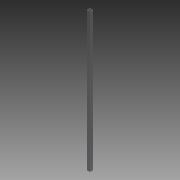
# Autodesk Inventor part: Square
Saved by Autodesk Inventor 2015 SP1 (Build 190203100, 203)
## iProperties
Created: 2015-02-01
Part Number: Square
Material: Aluminum
Document SubType Name: Modeling
Designer: Brian
Density: 2.7 g/cm^3
Appearance: Semi-Polished
Author: Brian
Autodesk Inventor part; units mm, degrees
ref_plane "YZ Plane" through (0, 0, 0) normal (1, 0, 0) x (0, 1, 0)
ref_plane "XZ Plane" through (0, 0, 0) normal (0, 1, 0) x (-1, 0, 0)
ref_plane "XY Plane" through (0, 0, 0) normal (0, 0, 1) x (1, 0, 0)
sketch "Sketch1" plane through (0, 0, 0) normal (0, 1, 0) x (-1, 0, 0)
  line L0 (12.7, -12.7) -> (-12.7, -12.7)
  line L1 (-12.7, -12.7) -> (-12.7, 12.7)
  line L2 (-12.7, 12.7) -> (12.7, 12.7)
  line L3 (12.7, 12.7) -> (12.7, -12.7)
  line L4 (-11.1125, -11.1125) -> (11.1125, -11.1125)
  line L5 (11.1125, -11.1125) -> (11.1125, 11.1125)
  line L6 (11.1125, 11.1125) -> (-11.1125, 11.1125)
  line L7 (-11.1125, 11.1125) -> (-11.1125, -11.1125)
  point P0 (0, 0)
  point P1 (0, -12.7)
  point P2 (-12.7, 0)
  dimension "d0" = 25.4
  dimension "d1" = 1.5875
  constraints: 16 end point, 4 parallel, 3 perpendicular, 2 midpoint, 1 horizontal, 1 horizontal alignment, 1 vertical alignment, 3 other
  measures "d0" distance of L0.start L0.end
  measures "d1" distance between parallel lines of L0 L4
extrude "Extrusion1" add sketch "Sketch1" along normal blind 1168.4
sketch "Sketch3" plane through (-12.7, 0, 12.7) normal (-1, 0, 0) x (0, 0, 1)
  arc A0 (-169.799, 314.325) -> (-166.624, 311.15) centre (-166.624, 314.325) ccw construction
  line L0 (-166.624, 311.15) -> (4.826, 311.15) construction
  arc A1 (4.826, 311.15) -> (8.001, 314.325) centre (4.826, 314.325) ccw construction
  line L1 (8.001, 314.325) -> (8.001, 442.976) construction
  arc A2 (8.001, 442.976) -> (4.826, 446.151) centre (4.826, 442.976) ccw construction
  line L2 (4.826, 446.151) -> (-32.4164, 446.151) construction
  arc A3 (-32.4164, 446.151) -> (-34.2128, 445.5939) centre (-32.4164, 442.976) ccw construction
  line L3 (-34.2128, 445.5939) -> (-168.4205, 353.498) construction
  arc A4 (-168.4205, 353.498) -> (-169.799, 350.8801) centre (-166.624, 350.8801) ccw construction
  line L4 (-169.799, 350.8801) -> (-169.799, 314.325) construction
  circle A5 centre (-12.7, 433.451) radius 3.3655 projected
  circle A6 centre (-12.7, 382.651) radius 3.3655 projected
  circle A7 centre (-12.7, 331.851) radius 3.3655 projected
  circle A8 centre (-63.5, 331.851) radius 3.3655 construction
  circle A9 centre (-114.3, 331.851) radius 3.3655 construction
  circle A10 centre (-165.1, 331.851) radius 3.3655 construction
  arc A11 (-169.799, 871.474) -> (-166.624, 868.299) centre (-166.624, 871.474) ccw construction
  line L5 (-166.624, 868.299) -> (4.826, 868.299) construction
  arc A12 (4.826, 868.299) -> (8.001, 871.474) centre (4.826, 871.474) ccw construction
  line L6 (8.001, 871.474) -> (8.001, 1000.125) construction
  arc A13 (8.001, 1000.125) -> (4.826, 1003.3) centre (4.826, 1000.125) ccw construction
  line L7 (4.826, 1003.3) -> (-32.4164, 1003.3) construction
  arc A14 (-32.4164, 1003.3) -> (-34.2128, 1002.7429) centre (-32.4164, 1000.125) ccw construction
  line L8 (-34.2128, 1002.7429) -> (-168.4205, 910.647) construction
  arc A15 (-168.4205, 910.647) -> (-169.799, 908.0291) centre (-166.624, 908.0291) ccw construction
  line L9 (-169.799, 908.0291) -> (-169.799, 871.474) construction
  circle A16 centre (-12.7, 990.6) radius 3.3655 projected
  circle A17 centre (-12.7, 939.8) radius 3.3655 projected
  circle A18 centre (-12.7, 889) radius 3.3655 projected
  circle A19 centre (-63.5, 889) radius 3.3655 construction
  circle A20 centre (-114.3, 889) radius 3.3655 construction
  circle A21 centre (-165.1, 889) radius 3.3655 construction
  circle A22 centre (-12.7, 1155.7) radius 3.3655
  point P0 (-12.7, 0)
  dimension "d7" = 165.1
  constraints: 1 centre point, 1 equal radius, 1 vertical alignment
  measures "d7" distance of A16.centre A22.centre
extrude "Extrusion2" cut sketch "Sketch3" against normal blind 25.4
body "Solid1"
